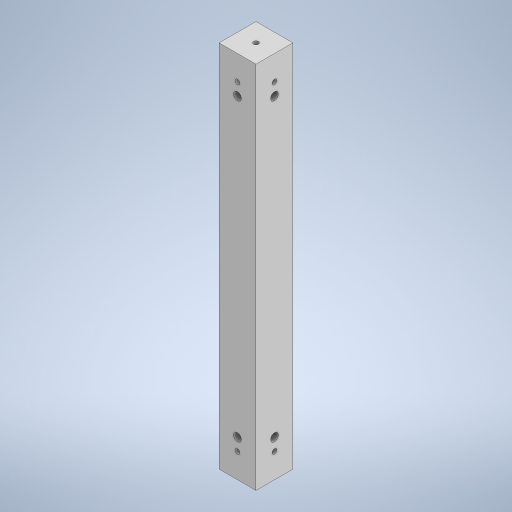
# Autodesk Inventor part: tensegrity_bar_4c
Saved by Autodesk Inventor 2023 (Build 270158000, 158)
## iProperties
Created: 2023-11-10
Part Number: tensegrity_bar_4c
Material: Všeobecné
Document SubType Name: Modeling
Designer: zavrel
Density: 1 g/cm^3
Appearance: Výchozí
Author: zavrel
Autodesk Inventor part; units mm, degrees
ref_plane "YZ Plane" through (0, 0, 0) normal (1, 0, 0) x (0, 1, 0)
ref_plane "XZ Plane" through (0, 0, 0) normal (0, 1, 0) x (-1, 0, 0)
ref_plane "XY Plane" through (0, 0, 0) normal (0, 0, 1) x (1, 0, 0)
sketch "Náčrt1" plane through (0, 0, 0) normal (0, 1, 0) x (-1, 0, 0)
  line L0 (0, 0) -> (15, 0)
  line L1 (15, 0) -> (15, -15)
  line L2 (15, -15) -> (0, -15)
  line L3 (0, -15) -> (0, 0)
  dimension "d0" = 15
  constraints: 8 end point, 2 parallel, 2 perpendicular, 1 horizontal
  measures "d0" distance of L0.end L1.end
extrude "Vysunutí1" add sketch "Náčrt1" along normal blind 150
sketch "Náčrt2" plane through (0, 150, 0) normal (0, 1, 0) x (1, 0, 0)
  line L0 (0, 15) -> (-15, 15) projected
  line L1 (-15, 15) -> (-15, 0) projected
  line L2 (-15, 0) -> (0, 0) projected
  line L3 (0, 0) -> (0, 15) projected
  circle A0 centre (-7.5, 7.5) radius 1
  line L4 (-15, 0) -> (0, 15) construction
  line L5 (-15, 15) -> (0, 0) construction
  point P0 (-7.5, 7.5)
  dimension "d3" = 2
  constraints: 4 end point, 1 centre point, 1 coincident, 1 midpoint, 1 perpendicular
  measures "d3" diameter of A0
extrude "Vysunutí2" cut sketch "Náčrt2" against normal through all contours A0
sketch "Náčrt3" plane through (0, 0, 0) normal (1, 0, 0) x (0, 0, -1)
  line L0 (0, 0) -> (15, 0) projected
  line L1 (15, 0) -> (15, 150) projected
  line L2 (0, 150) -> (15, 150) projected
  line L3 (0, 0) -> (0, 150) projected
  line L4 (7.5, 150) -> (7.5, 0) construction
  line L5 (15, 0) -> (0, 0) construction
  circle A0 centre (7.5, 135) radius 1.6
  circle A1 centre (7.5, 15) radius 1.6
  circle A2 centre (7.5, 140) radius 1
  circle A3 centre (7.5, 10) radius 1
  dimension "d6" = 3.2
  dimension "d7" = 15
  dimension "d8" = 15
  dimension "d16" = 2
  dimension "d17" = 10
  dimension "d18" = 10
  constraints: 4 centre point, 4 point on line, 2 end point, 2 equal radius, 2 midpoint
  measures "d6" diameter of A0
  measures "d7" distance from line of L2 A0.centre
  measures "d8" distance from line of L0 A1.centre
  measures "d16" diameter of A2
  measures "d17" distance from line of L2 A2.centre
  measures "d18" distance from line of L0 A3.centre
extrude "Vysunutí3" cut sketch "Náčrt3" against normal through all contours A0 | A1 | A2 | A3
sketch "Náčrt4" plane through (-15, 0, 0) normal (0, 0, 1) x (1, 0, 0)
  line L0 (0, 0) -> (15, 0) projected
  line L1 (15, 0) -> (15, 150) projected
  line L2 (0, 150) -> (15, 150) projected
  line L3 (0, 0) -> (0, 150) projected
  line L4 (6.5, 150) -> (8.5, 150) construction
  line L5 (7.5, 150) -> (7.5, 0) construction
  line L6 (8.5, 0) -> (6.5, 0) construction
  circle A0 centre (7.5, 135) radius 1.6
  circle A1 centre (7.5, 15) radius 1.6
  circle A2 centre (7.5, 140) radius 1
  circle A3 centre (7.5, 10) radius 1
  dimension "d11" = 3.2
  dimension "d12" = 15
  dimension "d13" = 15
  dimension "d19" = 2
  dimension "d20" = 10
  dimension "d21" = 10
  constraints: 4 centre point, 4 point on line, 2 end point, 2 equal radius, 2 midpoint
  measures "d11" diameter of A0
  measures "d12" distance from line of L2 A0.centre
  measures "d13" distance from line of L0 A1.centre
  measures "d19" diameter of A2
  measures "d20" distance from line of L2 A2.centre
  measures "d21" distance from line of L0 A3.centre
extrude "Vysunutí4" cut sketch "Náčrt4" against normal through all contours A0 | A1 | A2 | A3
